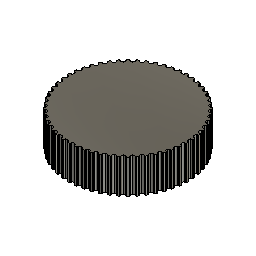
gear_56z (Autodesk Fusion 360 design; units mm, degrees)
Autodesk Fusion 360 part; units mm, degrees
sketch "Sketch1" plane through (0, 0, 0) normal (0, 0, 1) x (1, 0, 0) in component "gt2 pulley"
  circle A0 centre (0, 0) radius 17.8254 construction
  circle A1 centre (0, 0) radius 16.8214 construction
  line L0 (0, 0) -> (0, 17.8254) construction
  line L1 (0, 0) -> (0.9995, 17.7973) construction
  line L2 (0, 0) -> (1.4066, 17.7698) construction
  circle A2 centre (0, 0) radius 17.5714 construction
  arc A3 (0.3901, 17.4323) -> (0.4601, 17.1401) centre (1.3866, 17.5166) ccw
  circle A4 centre (0, 0) radius 17.4214 construction
  arc A5 (0.2426, 17.5697) -> (0, 17.5714) centre (0, 0) ccw
  arc A6 (0.3901, 17.4323) -> (0.2426, 17.5697) centre (0.2406, 17.4197) ccw
  arc A7 (0.4601, 17.1401) -> (0.9432, 16.7949) centre (0.9743, 17.349) ccw
  arc A8 (0, 17.5714) -> (-0.2426, 17.5697) centre (0, 0) ccw
  arc A9 (-0.2426, 17.5697) -> (-0.3901, 17.4323) centre (-0.2406, 17.4197) ccw
  arc A10 (-0.4601, 17.1401) -> (-0.3901, 17.4323) centre (-1.3866, 17.5166) ccw
  arc A11 (-0.9426, 16.7949) -> (-0.4601, 17.1401) centre (-0.9743, 17.349) ccw
  arc A12 (0.9432, 16.7949) -> (-0.9432, 16.7949) centre (0, 0) ccw
  point P0 (1.3866, 17.5166)
  point P1 (0, 17.5714)
  dimension "d18" = 35.6507
  dimension "d19" = 3.214
  dimension "d22" = 1.004
  dimension "d24" = 0.75
  dimension "d26" = 1
  dimension "d27" = 0.15
  dimension "d28" = 0.15
  dimension "d47" = 0.555
  dimension "d52" = 3.812
  constraint coincident A0.centre A1.centre
  constraint coincident A0 L0.end
  constraint vertical L0
  constraint coincident A0 L1.end
  constraint coincident A0 L2.end
  constraint concentric A1 A2
  constraint coincident A1 A7.end
  constraint coincident L1 A7.end
  constraint coincident A2 P0
  constraint coincident L2 P0
  constraint coincident P0 A3.centre
  constraint coincident A2 P1
  constraint coincident L0 P1
  constraint concentric A2 A4
  constraint coincident P1 A5.end
  constraint coincident A4 A6.centre
  constraint coincident A3.start A6.start
  constraint tangent A3 A6
  constraint tangent A3 A7
  constraint symmetric L0 A7.end A12.end
  constraint symmetric L0 A3.start A9.end
  constraint symmetric L0 A3.end A10.start
  constraint symmetric L0 A3 A10
  constraint symmetric L0 A5.start A8.end
  constraint symmetric L0 P1 A5.end
  constraint symmetric L0 A5 A8
  constraint symmetric L0 A6 A9
  constraint symmetric L0 A7 A11
  constraint coincident A1 A11.start
  constraint tangent A1 A7
  constraint coincident L1 A7.centre
  measures "d18" diameter of A0
  measures "d19" angle of L0 L1
  measures "d22" distance of A0 A1
  measures "d24" distance of A1 A2
  measures "d26" radius of A3
  measures "d27" distance of A2 A4
  measures "d28" radius of A6
  measures "d47" radius of A7
extrude "Extrude1" add sketch "Sketch1" along normal blind 7 makes body 1
pattern_circular "C-Pattern1" count 56 over 360 about axis through (0, 0, 1.75) along (0, 0, 1) of bodies 1 makes body 2 at (-1.9872, 16.7036, 4.6667) makes body 3 at (-3.8449, 16.376, 4.6667) makes body 4 at (-4.8578, 16.1046, 2.3333) makes body 5 at (-7.9522, 14.823, 4.6667) makes body 6 at (-9.0378, 14.1872, 4.6667) makes body 7 at (-10.5695, 13.086, 4.6667) makes body 8 at (-12.4016, 11.3647, 4.6667) makes body 9 at (-13.2164, 10.406, 4.6667) makes body 10 at (-14.2984, 8.8608, 4.6667) makes body 11 at (-15.4592, 6.631, 4.6667) makes body 12 at (-15.9116, 5.457, 4.6667) makes body 13 at (-16.4225, 3.6411, 4.6667) makes body 14 at (-16.7818, 1.153, 4.6667) makes body 15 at (-16.8053, 0.7338, 2.3333) makes body 16 at (-16.7036, -1.9872, 4.6667) makes body 17 at (-16.376, -3.8449, 4.6667) makes body 18 at (-15.6201, -6.2425, 4.6667) makes body 19 at (-15.1099, -7.3925, 4.6667) makes body 20 at (-14.6199, -8.3197, 2.3333) makes body 21 at (-12.6818, -11.0512, 4.6667) makes body 22 at (-11.3647, -12.4016, 4.6667) makes body 23 at (-11.0517, -12.6814, 2.3333) makes body 24 at (-8.8608, -14.2984, 4.6667) makes body 25 at (-7.9527, -14.8227, 2.3333) makes body 26 at (-6.2431, -15.6199, 2.3333) makes body 27 at (-3.0247, -16.5472, 4.6667) makes body 28 at (-1.7795, -16.727, 4.6667) makes body 29 at (-0.7338, -16.8053, 2.3333) makes body 30 at (1.9872, -16.7036, 4.6667) makes body 31 at (3.0241, -16.5473, 2.3333) makes body 32 at (5.6543, -15.8426, 4.6667) makes body 33 at (7.9522, -14.823, 4.6667) makes body 34 at (8.3197, -14.6199, 2.3333) makes body 35 at (11.0512, -12.6818, 4.6667) makes body 36 at (12.4016, -11.3647, 4.6667) makes body 37 at (13.2164, -10.406, 4.6667) makes body 38 at (14.2984, -8.8608, 4.6667) makes body 39 at (15.2006, -7.2042, 4.6667) makes body 40 at (15.6199, -6.2431, 2.3333) makes body 41 at (16.4225, -3.6411, 4.6667) makes body 42 at (16.727, -1.7795, 4.6667) makes body 43 at (16.8053, -0.7338, 2.3333) makes body 44 at (16.7036, 1.9872, 4.6667) makes body 45 at (16.2209, 4.4544, 4.6667) makes body 46 at (15.8426, 5.6543, 4.6667) makes body 47 at (15.1099, 7.3925, 4.6667) makes body 48 at (14.6199, 8.3197, 2.3333) makes body 49 at (13.086, 10.5695, 4.6667) makes body 50 at (11.3647, 12.4016, 4.6667) makes body 51 at (10.406, 13.2164, 4.6667) makes body 52 at (8.3202, 14.6196, 4.6667) makes body 53 at (6.631, 15.4592, 4.6667) makes body 54 at (4.8584, 16.1045, 4.6667) makes body 55 at (3.6411, 16.4225, 4.6667) makes body 56 at (2.6108, 16.6175, 2.3333)
sketch "Sketch2" plane through (0, 0, 7) normal (0, 0, 1) x (-1, 0, 0)
  arc A0 (-14.9679, -8.9442) -> (-15.0058, -9.1422) centre (-14.8777, -9.0641) ccw
  arc A1 (-15.0058, -9.1422) -> (-14.7476, -9.5531) centre (0, 0) ccw
  arc A2 (-14.7476, -9.5531) -> (-14.5528, -9.6049) centre (-14.6216, -9.4716) ccw
  arc A3 (-14.2681, -9.5087) -> (-14.5528, -9.6049) centre (-14.094, -10.4934) ccw
  arc A4 (-13.7192, -9.7336) -> (-14.2681, -9.5087) centre (-14.1715, -10.0552) ccw
  arc A5 (-14.7224, -8.1368) -> (-13.7192, -9.7336) centre (0, 0) ccw
  arc A6 (-14.7577, -8.7294) -> (-14.7224, -8.1368) centre (-15.2082, -8.4053) ccw
  arc A7 (-14.9679, -8.9442) -> (-14.7577, -8.7294) centre (-15.5694, -8.1453) ccw
  circle A8 centre (0, 0) radius 16.8214
  constraint concentric A1 A8
extrude "Extrude2" add sketch "Sketch2" against normal blind 7 contours A5 A8 bodies 1 2 3 4 5 6 7 8 9 10 11 12 13 14 15 16 17 18 19 20 21 22 23 24 25 26 27 28 29 30 31 32 33 34 35 36 37 38 39 40 41 42 43 44 45 46 47 48 49 50 51 52 53 54 55 56
extrude "Extrude3" add 1 faces at (6.6266, -8.8142, 7) along direction (0, 0, 1) blind 3 on bodies 1 bodies 1
extrude "Extrude4" [suppressed] in component "gt2 pulley"
pattern_circular "C-Pattern7" [suppressed] in component "gt2 pulley"
extrude "Extrude3'" [suppressed] in component "gt2 pulley"
pattern_circular "C-Pattern6" [suppressed] in component "gt2 pulley"
extrude "Extrude2'" [suppressed] in component "gt2 pulley"
pattern_circular "C-Pattern5" [suppressed] in component "gt2 pulley"
extrude "Extrude1'" [suppressed] in component "gt2 pulley"
pattern_circular "C-Pattern4" [suppressed] in component "gt2 pulley"
pattern_circular "C-Pattern3" [suppressed] in component "gt2 pulley"
pattern_circular "C-Pattern2" [suppressed] in component "gt2 pulley"
pattern_circular "C-Pattern1'" [suppressed] in component "gt2 pulley"
copy_body "Body->Comp1" [suppressed] in component "Component"
copy_body "Body->Comp2" [suppressed] in component "Component'"
copy_body "Body->Comp3" [suppressed] in component "Component''"
copy_body "Body->Comp4" [suppressed] in component "Component'''"
copy_body "Body->Comp5" [suppressed] in component "Component''''"
copy_body "Body->Comp6" [suppressed] in component "Component'''''"
copy_body "Body->Comp7" [suppressed] in component "Component''''''"
copy_body "Body->Comp8" [suppressed] in component "Component'''''''"
copy_body "Body->Comp9" [suppressed] in component "Component''''''''"
copy_body "Body->Comp10" [suppressed] in component "Component'''''''''"
copy_body "Body->Comp11" [suppressed] in component "Component''''''''''"
copy_body "Body->Comp12" [suppressed] in component "Component'''''''''''"
copy_body "Body->Comp13" [suppressed] in component "Component''''''''''''"
copy_body "Body->Comp14" [suppressed] in component "Component'''''''''''''"
copy_body "Body->Comp15" [suppressed] in component "Component''''''''''''''"
copy_body "Body->Comp16" [suppressed] in component "Component'''''''''''''''"
copy_body "Body->Comp17" [suppressed] in component "Component''''''''''''''''"
copy_body "Body->Comp18" [suppressed] in component "Component'''''''''''''''''"
copy_body "Body->Comp19" [suppressed] in component "Component''''''''''''''''''"
copy_body "Body->Comp20" [suppressed] in component "Component'''''''''''''''''''"
component "gt2 pulley" placed x (1, 0, 0) y (0, 1, 0) z (0, 0, 1) at (0, 0, 0)
equation "NumTeeth = 56" comment "min 20"
equation "ToothPitch = 2 mm"
equation "PullyDia = NumTeeth * ToothPitch / PI"
equation "ToothAng = ( ( 360 / NumTeeth ) * 1 deg )"
equation "TransOffsetAngle = ToothAng * 0.2"
equation "Sholulder_Radius = 0.15 mm"
equation "Root_Radius = 0.555 mm"
equation "TransRadius = 1 mm"
equation "ToolHeight = 0.75 mm"
equation "PLD = 0.254 mm"
equation "d18 = PullyDia"
equation "d19 = ToothAng / 2"
equation "d22 = PLD + ToolHeight"
equation "d24 = ToolHeight"
equation "d26 = TransRadius"
equation "d27 = Sholulder_Radius"
equation "d31 = NumTeeth"
equation "d33 = NumTeeth"
equation "d35 = NumTeeth"
equation "d37 = NumTeeth"
equation "d41 = NumTeeth"
equation "d45 = NumTeeth"
equation "d47 = Root_Radius"
equation "d50 = NumTeeth"
equation "d55 = NumTeeth"
